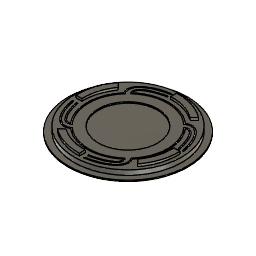
button (Autodesk Fusion 360 design; units mm, degrees)
Autodesk Fusion 360 part; units mm, degrees
note: some values were not read from the file. Set by a fixed rule: which sketch regions a step uses.
sketch "Sketch8" plane through (0, 0, 0) normal (0, 0, 1) x (1, 0, 0)
  circle A0 centre (0, 0) radius 40
  circle A1 centre (-48, 0) radius 2
  circle A2 centre (-48, 0) radius 4
  circle A3 centre (0, 0) radius 48 construction
  line L0 (-39.5395, 39.5395) -> (0, 0) construction
  line L1 (0, 0) -> (-68, 0) construction
  line L2 (-49.7486, 0.9707) -> (-47.9713, 22.4598) construction
  line L3 (-47.9713, 22.4598) -> (-35.9328, 37.1294) construction
  line L4 (-35.9328, 37.1294) -> (-26.8347, 29.6631) construction
  spline S0 degree 3 poles (-49.7486, 0.9707) (-47.9713, 22.4598) (-35.9328, 37.1294) (-26.8347, 29.6631) knots 0 0 0 0 1 1 1 1
  line L5 (-47.2849, 1.8678) -> (-43.4766, 23.129) construction
  line L6 (-43.4766, 23.129) -> (-35.7051, 32.0803) construction
  line L7 (-35.7051, 32.0803) -> (-29.6631, 26.8347) construction
  spline S1 degree 3 poles (-47.2849, 1.8678) (-43.4766, 23.129) (-35.7051, 32.0803) (-29.6631, 26.8347) knots 0 0 0 0 1 1 1 1
  dimension "d92" = 80
  dimension "d93" = 4
  dimension "d94" = 2
  dimension "d95" = 8
  dimension "d96" = 68
  dimension "d97" = 45
  dimension "d100" = 4
  dimension "d101" = 90
  dimension "d102" = 90
  dimension "d103" = 5.0542
  dimension "d104" = 2
  constraint coincident A0.centre A3.centre
  constraint horizontal A0.centre A1.centre
  constraint coincident A1.centre A3
  constraint horizontal L1
  constraint coincident A0 L7.end
  constraint coincident A0 L4.end
  constraint coincident A1 L2.start
  constraint coincident A1 L5.start
  constraint coincident A3 L6.end
  measures "d92" diameter of A0
  measures "d93" diameter of A1
  measures "d94" distance of A1
  measures "d96" distance of A0.centre L1.end
  measures "d97" angle of L0 L1
  measures "d100" distance of L4.end L7.end
  measures "d101" angle of L3 L4
  measures "d102" angle of L6 L7
  measures "d103" distance of L3.end L6.end
  measures "d104" distance of L0 L7.end
extrude "Extrude11" add sketch "Sketch8" along normal blind 6 contours A0 makes body 1
extrude "Extrude16" add sketch "Sketch8" along normal blind 6 separate body contours A0 A2 S0 S1 makes body 2
extrude "Extrude18" add sketch "Sketch8" along normal blind 6 contours A1 A2 S0 S1 | A1 A2 S0 S1 | A1 bodies 2
pattern_circular "C-Pattern2" count 4 over 360 about axis through (0, 0, 1.75) along (0, 0, 1) of "Extrude16", "Extrude18" makes body 3 at (-6.6102, -49.0265, 2) makes body 4 at (49.0265, -6.6102, 2) makes body 5 at (9.3884, 48.4723, 4)
sketch "Sketch11" plane through (0, 0, 6) normal (0, 0, 1) x (-1, 0, 0)
  circle A0 centre (0, 0) radius 40
  circle A1 centre (0, 0) radius 38
  dimension "d126" = 76
  constraint concentric A0 A1
  measures "d126" diameter of A1
sketch "Sketch15" plane through (0, 0, 0) normal (0, 0, -1) x (1, 0, 0)
  circle A0 centre (0, 0) radius 40
  circle A1 centre (0, 0) radius 54.5
  circle A2 centre (0, 0) radius 41.2
  spline S0 degree 3 poles (3.7237, -49.461) (23.6891, -46.9339) (36.806, -35.5387) (29.6631, -26.8347) knots 0.043317 0.043317 0.043317 0.043317 1 1 1 1
  spline S1 degree 3 poles (3.8491, -46.9116) (23.6813, -42.9865) (31.9143, -35.5139) (26.8347, -29.6631) knots 0.031644 0.031644 0.031644 0.031644 1 1 1 1
  spline S2 degree 3 poles (46.9116, 3.8491) (42.9865, 23.6813) (35.5139, 31.9143) (29.6631, 26.8347) knots 0.031644 0.031644 0.031644 0.031644 1 1 1 1
  spline S3 degree 3 poles (49.461, 3.7237) (46.9339, 23.6891) (35.5387, 36.806) (26.8347, 29.6631) knots 0.043317 0.043317 0.043317 0.043317 1 1 1 1
  arc A3 (46.9116, 3.8491) -> (49.461, 3.7237) centre (48, 0) ccw
  spline S4 degree 3 poles (3.8491, -46.9116) (23.6813, -42.9865) (31.9143, -35.5139) (26.8347, -29.6631) knots 0.031644 0.031644 0.031644 0.031644 1 1 1 1
  arc A4 (3.8491, -46.9116) -> (3.7237, -49.461) centre (0, -48) ccw
  spline S5 degree 3 poles (3.7237, -49.461) (23.6891, -46.9339) (36.806, -35.5387) (29.6631, -26.8347) knots 0.043317 0.043317 0.043317 0.043317 1 1 1 1
  arc A5 (26.8347, -29.6631) -> (29.6631, -26.8347) centre (0, 0) ccw
  arc A6 (-46.9116, -3.8491) -> (-49.461, -3.7237) centre (-48, 0) ccw
  spline S6 degree 3 poles (-46.9116, -3.8491) (-42.9865, -23.6813) (-35.5139, -31.9143) (-29.6631, -26.8347) knots 0.031644 0.031644 0.031644 0.031644 1 1 1 1
  spline S7 degree 3 poles (-49.461, -3.7237) (-46.9339, -23.6891) (-35.5387, -36.806) (-26.8347, -29.6631) knots 0.043317 0.043317 0.043317 0.043317 1 1 1 1
  spline S8 degree 3 poles (-3.7237, 49.461) (-23.6891, 46.9339) (-36.806, 35.5387) (-29.6631, 26.8347) knots 0.043317 0.043317 0.043317 0.043317 1 1 1 1
  spline S9 degree 3 poles (-3.8491, 46.9116) (-23.6813, 42.9865) (-31.9143, 35.5139) (-26.8347, 29.6631) knots 0.031644 0.031644 0.031644 0.031644 1 1 1 1
  arc A7 (-3.8491, 46.9116) -> (-3.7237, 49.461) centre (0, 48) ccw
  arc A8 (-2.6359, 43.5347) -> (-3.3902, 43.6926) centre (-3.2459, 42.5013) ccw
  arc A9 (-5.0161, 50.5234) -> (-4.2204, 51.0125) centre (-5.1971, 51.7097) ccw
  arc A10 (44.9096, 4.1704) -> (45.3659, 5.3977) centre (44.1951, 5.1345) ccw
  arc A11 (50.4825, 5.0583) -> (50.9808, 4.2495) centre (51.6699, 5.2319) ccw
  arc A12 (5.0569, -50.486) -> (4.2495, -50.9837) centre (5.2316, -51.6732) ccw
  arc A13 (4.1719, -44.9087) -> (5.3984, -45.3653) centre (5.1361, -44.1943) ccw
  spline S10 degree 3 poles (-50.566, -4.5228) (-49.2121, -14.4065) (-45.7541, -22.6133) (-41.369, -27.6472) (-39.0131, -30.3518) (-36.3616, -32.1693) (-33.542, -32.6861) (-31.191, -33.1171) (-28.7542, -32.5715) (-26.5965, -30.9961) (-26.4205, -30.8676) (-26.2461, -30.7325) (-26.0734, -30.5907) knots 0.053517 0.053517 0.053517 0.053517 0.521659 0.521659 0.521659 0.77317 0.77317 0.77317 0.982893 0.982893 0.982893 1 1 1 1
  arc A14 (-45.5388, -4.5807) -> (-50.566, -4.5228) centre (-48, 0) ccw
  spline S11 degree 3 poles (-45.5388, -4.5807) (-43.7792, -13.0486) (-41.3441, -19.2391) (-38.8101, -22.9312) (-37.3314, -25.0858) (-35.8297, -26.3571) (-34.5346, -26.8443) (-33.5151, -27.2279) (-32.632, -27.1972) (-31.6708, -26.744) (-31.2743, -26.557) (-30.8658, -26.2897) (-30.4498, -25.9285) knots 0.04768 0.04768 0.04768 0.04768 0.474261 0.474261 0.474261 0.723202 0.723202 0.723202 0.919177 0.919177 0.919177 1 1 1 1
  spline S12 degree 3 poles (-4.5807, 45.5388) (-13.0486, 43.7792) (-19.2391, 41.3441) (-22.9312, 38.8101) (-25.0858, 37.3314) (-26.3571, 35.8297) (-26.8443, 34.5346) (-27.2279, 33.5151) (-27.1972, 32.632) (-26.744, 31.6708) (-26.557, 31.2743) (-26.2897, 30.8658) (-25.9285, 30.4498) knots 0.04768 0.04768 0.04768 0.04768 0.474261 0.474261 0.474261 0.723202 0.723202 0.723202 0.919177 0.919177 0.919177 1 1 1 1
  arc A15 (-4.5807, 45.5388) -> (-4.5228, 50.566) centre (0, 48) ccw
  spline S13 degree 3 poles (-4.5228, 50.566) (-14.4065, 49.2121) (-22.6133, 45.7541) (-27.6472, 41.369) (-30.3518, 39.0131) (-32.1693, 36.3616) (-32.6861, 33.542) (-33.1171, 31.191) (-32.5715, 28.7542) (-30.9961, 26.5965) (-30.8676, 26.4205) (-30.7325, 26.2461) (-30.5907, 26.0734) knots 0.053517 0.053517 0.053517 0.053517 0.521659 0.521659 0.521659 0.77317 0.77317 0.77317 0.982893 0.982893 0.982893 1 1 1 1
  spline S14 degree 3 poles (45.5388, 4.5807) (43.7792, 13.0486) (41.3441, 19.2391) (38.8101, 22.9312) (37.3314, 25.0858) (35.8297, 26.3571) (34.5346, 26.8443) (33.5151, 27.2279) (32.632, 27.1972) (31.6708, 26.744) (31.2743, 26.557) (30.8658, 26.2897) (30.4498, 25.9285) knots 0.04768 0.04768 0.04768 0.04768 0.474261 0.474261 0.474261 0.723202 0.723202 0.723202 0.919177 0.919177 0.919177 1 1 1 1
  arc A16 (45.5388, 4.5807) -> (50.566, 4.5228) centre (48, 0) ccw
  spline S15 degree 3 poles (50.566, 4.5228) (49.2121, 14.4065) (45.7541, 22.6133) (41.369, 27.6472) (39.0131, 30.3518) (36.3616, 32.1693) (33.542, 32.6861) (31.191, 33.1171) (28.7542, 32.5715) (26.5965, 30.9961) (26.4205, 30.8676) (26.2461, 30.7325) (26.0734, 30.5907) knots 0.053517 0.053517 0.053517 0.053517 0.521659 0.521659 0.521659 0.77317 0.77317 0.77317 0.982893 0.982893 0.982893 1 1 1 1
  spline S16 degree 3 poles (4.5228, -50.566) (14.4065, -49.2121) (22.6133, -45.7541) (27.6472, -41.369) (30.3518, -39.0131) (32.1693, -36.3616) (32.6861, -33.542) (33.1171, -31.191) (32.5715, -28.7542) (30.9961, -26.5965) (30.8676, -26.4205) (30.7325, -26.2461) (30.5907, -26.0734) knots 0.053517 0.053517 0.053517 0.053517 0.521659 0.521659 0.521659 0.77317 0.77317 0.77317 0.982893 0.982893 0.982893 1 1 1 1
  arc A17 (4.5807, -45.5388) -> (4.5228, -50.566) centre (0, -48) ccw
  spline S17 degree 3 poles (4.5807, -45.5388) (13.0486, -43.7792) (19.2391, -41.3441) (22.9312, -38.8101) (25.0858, -37.3314) (26.3571, -35.8297) (26.8443, -34.5346) (27.2279, -33.5151) (27.1972, -32.632) (26.744, -31.6708) (26.557, -31.2743) (26.2897, -30.8658) (25.9285, -30.4498) knots 0.04768 0.04768 0.04768 0.04768 0.474261 0.474261 0.474261 0.723202 0.723202 0.723202 0.919177 0.919177 0.919177 1 1 1 1
  dimension "d155" = 109
  dimension "d156" = 82.4
  dimension "d167" = 1.2
  dimension "d168" = 1.2
  dimension "d169" = 1.2
  dimension "d170" = 1.2
  dimension "d171" = 1.2
  dimension "d172" = 1.2
  dimension "d178" = 1.2
  dimension "d207" = 1.2
  dimension "d208" = 1.2
  constraint concentric A0 A1
  constraint concentric A0 A2
  measures "d155" diameter of A1
  measures "d156" diameter of A2
  measures "d167" radius of A8
  measures "d168" radius of A9
  measures "d169" radius of A10
  measures "d170" radius of A11
  measures "d171" radius of A12
  measures "d172" radius of A13
extrude "Extrude23" add sketch "Sketch15" against normal blind 6 separate body makes body 6
combine "Combine4" operation add target body 1 tool bodies 3 4 5 2 6 makes body 7 at (46.2947, 10.9613, 0)
sketch "Sketch18" plane through (0, 0, 6) normal (0, 0, 1) x (-1, 0, 0)
  spline S0 degree 3 poles (50.566, -4.5228) (49.2121, -14.4065) (45.7541, -22.6133) (41.369, -27.6472) (39.0131, -30.3518) (36.3616, -32.1693) (33.542, -32.6861) (31.2997, -33.0972) (28.9795, -32.6199) (26.8976, -31.2084) knots 0.053517 0.053517 0.053517 0.053517 0.521659 0.521659 0.521659 0.77317 0.77317 0.77317 0.97319 0.97319 0.97319 0.97319
  arc A0 (-31.4398, 26.6266) -> (-31.2084, -26.8976) centre (0, 0) ccw
  spline S1 degree 3 poles (31.4398, -26.6266) (31.5172, -26.6688) (31.5942, -26.7079) (31.6708, -26.744) (32.632, -27.1972) (33.5151, -27.2279) (34.5346, -26.8443) (35.8297, -26.3571) (37.3314, -25.0858) (38.8101, -22.9312) (41.3441, -19.2391) (43.7792, -13.0486) (45.5388, -4.5807) knots -0.934786 -0.934786 -0.934786 -0.934786 -0.919177 -0.919177 -0.919177 -0.723202 -0.723202 -0.723202 -0.474261 -0.474261 -0.474261 -0.04768 -0.04768 -0.04768 -0.04768
  arc A1 (50.566, -4.5228) -> (45.5388, -4.5807) centre (48, 0) ccw
  circle A2 centre (48, 0) radius 6
  circle A3 centre (0, 0) radius 54.5
  arc A4 (4.5228, 50.566) -> (4.5807, 45.5388) centre (0, 48) ccw
  spline S2 degree 3 poles (4.5228, 50.566) (14.4065, 49.2121) (22.6133, 45.7541) (27.6472, 41.369) (30.3518, 39.0131) (32.1693, 36.3616) (32.6861, 33.542) (33.0972, 31.2997) (32.6199, 28.9795) (31.2084, 26.8976) knots 0.053517 0.053517 0.053517 0.053517 0.521659 0.521659 0.521659 0.77317 0.77317 0.77317 0.97319 0.97319 0.97319 0.97319
  spline S3 degree 3 poles (26.6266, 31.4398) (26.6688, 31.5172) (26.7079, 31.5942) (26.744, 31.6708) (27.1972, 32.632) (27.2279, 33.5151) (26.8443, 34.5346) (26.3571, 35.8297) (25.0858, 37.3314) (22.9312, 38.8101) (19.2391, 41.3441) (13.0486, 43.7792) (4.5807, 45.5388) knots -0.934786 -0.934786 -0.934786 -0.934786 -0.919177 -0.919177 -0.919177 -0.723202 -0.723202 -0.723202 -0.474261 -0.474261 -0.474261 -0.04768 -0.04768 -0.04768 -0.04768
  spline S4 degree 3 poles (-4.9578, -50.5049) (-14.6472, -49.1102) (-22.6873, -45.6896) (-27.6472, -41.369) (-30.3518, -39.0131) (-32.1693, -36.3616) (-32.6861, -33.542) (-33.0972, -31.2997) (-32.6199, -28.9795) (-31.2084, -26.8976) knots 0.060402 0.060402 0.060402 0.060402 0.521659 0.521659 0.521659 0.77317 0.77317 0.77317 0.97319 0.97319 0.97319 0.97319
  spline S5 degree 3 poles (-31.4398, 26.6266) (-31.5172, 26.6688) (-31.5942, 26.7079) (-31.6708, 26.744) (-32.632, 27.1972) (-33.5151, 27.2279) (-34.5346, 26.8443) (-35.8297, 26.3571) (-37.3314, 25.0858) (-38.8101, 22.9312) (-41.2659, 19.3529) (-43.6289, 13.428) (-45.3742, 5.3575) knots -0.934786 -0.934786 -0.934786 -0.934786 -0.919177 -0.919177 -0.919177 -0.723202 -0.723202 -0.723202 -0.474261 -0.474261 -0.474261 -0.060835 -0.060835 -0.060835 -0.060835
  arc A5 (-45.3742, 5.3575) -> (-45.0133, 4.2567) centre (-44.1951, 5.1345) ccw
  arc A6 (-50.8748, 4.3331) -> (-45.0133, 4.2567) centre (-48, 0) ccw
  arc A7 (-50.8748, 4.3331) -> (-50.5094, 4.9263) centre (-51.6699, 5.2319) ccw
  spline S6 degree 3 poles (-50.5094, 4.9263) (-49.1175, 14.6298) (-45.6942, 22.6819) (-41.369, 27.6472) (-39.0131, 30.3518) (-36.3616, 32.1693) (-33.542, 32.6861) (-31.2997, 33.0972) (-28.9795, 32.6199) (-26.8976, 31.2084) knots 0.059903 0.059903 0.059903 0.059903 0.521659 0.521659 0.521659 0.77317 0.77317 0.77317 0.97319 0.97319 0.97319 0.97319
  arc A8 (26.6266, 31.4398) -> (-26.8976, 31.2084) centre (0, 0) ccw
  arc A9 (31.4398, -26.6266) -> (31.2084, 26.8976) centre (0, 0) ccw
  arc A10 (-26.6266, -31.4398) -> (26.8976, -31.2084) centre (0, 0) ccw
  spline S7 degree 3 poles (-26.6266, -31.4398) (-26.6688, -31.5172) (-26.7079, -31.5942) (-26.744, -31.6708) (-27.1972, -32.632) (-27.2279, -33.5151) (-26.8443, -34.5346) (-26.3571, -35.8297) (-25.0858, -37.3314) (-22.9312, -38.8101) (-19.2391, -41.3441) (-13.0486, -43.7792) (-4.5807, -45.5388) knots -0.934786 -0.934786 -0.934786 -0.934786 -0.919177 -0.919177 -0.919177 -0.723202 -0.723202 -0.723202 -0.474261 -0.474261 -0.474261 -0.04768 -0.04768 -0.04768 -0.04768
  arc A11 (-4.3245, -50.8876) -> (-4.5807, -45.5388) centre (0, -48) ccw
  arc A12 (-4.3245, -50.8876) -> (-4.9578, -50.5049) centre (-5.2316, -51.6732) ccw
  dimension "d185" = 12
  constraint concentric A1 A2
  measures "d185" diameter of A2
extrude "Extrude26" add sketch "Sketch18" against normal blind 6 contours S0 S1 A1 A2 | S0 S1 A1 A2 bodies 1 7
pattern_circular "C-Pattern5" count 4 over 360 about axis through (0, 0, 1.75) along (0, 0, 1) of "Extrude26"
sketch "Sketch19" plane through (0, 0, 6) normal (0, 0, 1) x (-1, 0, 0)
  spline S0 degree 3 poles (-46.5038, 5.8105) (-42.4857, 24.22) (-35.3171, 31.7435) (-29.6631, 26.8347) knots 0.064208 0.064208 0.064208 0.064208 1 1 1 1
  arc A0 (-29.6631, 26.8347) -> (-29.6631, -26.8347) centre (0, 0) ccw
  spline S1 degree 3 poles (-29.6631, -26.8347) (-36.5444, -35.2199) (-24.6228, -46.1028) (-5.8891, -49.1482) knots -1 -1 -1 -1 -0.078355 -0.078355 -0.078355 -0.078355
  spline S2 degree 3 poles (-5.8105, -46.5038) (-24.22, -42.4857) (-31.7435, -35.3171) (-26.8347, -29.6631) knots 0.064208 0.064208 0.064208 0.064208 1 1 1 1
  arc A1 (-26.8347, -29.6631) -> (26.8347, -29.6631) centre (0, 0) ccw
  spline S3 degree 3 poles (26.8347, -29.6631) (35.2199, -36.5444) (46.1028, -24.6228) (49.1482, -5.8891) knots -1 -1 -1 -1 -0.078355 -0.078355 -0.078355 -0.078355
  arc A2 (49.1482, -5.8891) -> (50.4263, -5.4875) centre (48, 0) ccw
  spline S4 degree 3 poles (50.4263, -5.4875) (48.9827, -14.9399) (45.6106, -22.778) (41.369, -27.6472) (39.0131, -30.3518) (36.3616, -32.1693) (33.542, -32.6861) (31.2997, -33.0972) (28.9795, -32.6199) (26.8976, -31.2084) knots 0.068835 0.068835 0.068835 0.068835 0.521659 0.521659 0.521659 0.77317 0.77317 0.77317 0.97319 0.97319 0.97319 0.97319
  circle A3 centre (0, 0) radius 54.5
  spline S5 degree 3 poles (31.4398, -26.6266) (31.5172, -26.6688) (31.5942, -26.7079) (31.6708, -26.744) (32.632, -27.1972) (33.5151, -27.2279) (34.5346, -26.8443) (35.8297, -26.3571) (37.3314, -25.0858) (38.8101, -22.9312) (41.2625, -19.3579) (43.6223, -13.4446) (45.3669, -5.3913) knots -0.934786 -0.934786 -0.934786 -0.934786 -0.919177 -0.919177 -0.919177 -0.723202 -0.723202 -0.723202 -0.474261 -0.474261 -0.474261 -0.061414 -0.061414 -0.061414 -0.061414
  arc A4 (45.3669, -5.3913) -> (46.5038, -5.8105) centre (48, 0) ccw
  spline S6 degree 3 poles (46.5038, -5.8105) (42.4857, -24.22) (35.3171, -31.7435) (29.6631, -26.8347) knots 0.064208 0.064208 0.064208 0.064208 1 1 1 1
  arc A5 (29.6631, -26.8347) -> (29.6631, 26.8347) centre (0, 0) ccw
  spline S7 degree 3 poles (29.6631, 26.8347) (36.5444, 35.2199) (24.6228, 46.1028) (5.8891, 49.1482) knots -1 -1 -1 -1 -0.078355 -0.078355 -0.078355 -0.078355
  arc A6 (5.3913, 45.3669) -> (5.8105, 46.5038) centre (0, 48) ccw
  arc A7 (-31.4398, 26.6266) -> (-31.2084, -26.8976) centre (0, 0) ccw
  spline S8 degree 3 poles (5.8105, 46.5038) (24.22, 42.4857) (31.7435, 35.3171) (26.8347, 29.6631) knots 0.064208 0.064208 0.064208 0.064208 1 1 1 1
  arc A8 (26.8347, 29.6631) -> (-26.8347, 29.6631) centre (0, 0) ccw
  spline S9 degree 3 poles (-26.8347, 29.6631) (-35.2199, 36.5444) (-46.1028, 24.6228) (-49.1482, 5.8891) knots -1 -1 -1 -1 -0.078355 -0.078355 -0.078355 -0.078355
  circle A9 centre (0, 0) radius 54.5
  circle A10 centre (0, 0) radius 60.5
  spline S10 degree 3 poles (26.6266, 31.4398) (26.6688, 31.5172) (26.7079, 31.5942) (26.744, 31.6708) (27.1972, 32.632) (27.2279, 33.5151) (26.8443, 34.5346) (26.3571, 35.8297) (25.0858, 37.3314) (22.9312, 38.8101) (19.3579, 41.2625) (13.4446, 43.6223) (5.3913, 45.3669) knots -0.934786 -0.934786 -0.934786 -0.934786 -0.919177 -0.919177 -0.919177 -0.723202 -0.723202 -0.723202 -0.474261 -0.474261 -0.474261 -0.061414 -0.061414 -0.061414 -0.061414
  spline S11 degree 3 poles (5.4875, 50.4263) (14.9399, 48.9827) (22.778, 45.6106) (27.6472, 41.369) (30.3518, 39.0131) (32.1693, 36.3616) (32.6861, 33.542) (33.0972, 31.2997) (32.6199, 28.9795) (31.2084, 26.8976) knots 0.068835 0.068835 0.068835 0.068835 0.521659 0.521659 0.521659 0.77317 0.77317 0.77317 0.97319 0.97319 0.97319 0.97319
  arc A11 (31.4398, -26.6266) -> (31.2084, 26.8976) centre (0, 0) ccw
  arc A12 (5.8891, 49.1482) -> (5.4875, 50.4263) centre (0, 48) ccw
  arc A13 (-26.6266, -31.4398) -> (26.8976, -31.2084) centre (0, 0) ccw
  spline S12 degree 3 poles (-5.4875, -50.4263) (-14.9399, -48.9827) (-22.778, -45.6106) (-27.6472, -41.369) (-30.3518, -39.0131) (-32.1693, -36.3616) (-32.6861, -33.542) (-33.0972, -31.2997) (-32.6199, -28.9795) (-31.2084, -26.8976) knots 0.068835 0.068835 0.068835 0.068835 0.521659 0.521659 0.521659 0.77317 0.77317 0.77317 0.97319 0.97319 0.97319 0.97319
  spline S13 degree 3 poles (-31.4398, 26.6266) (-31.5172, 26.6688) (-31.5942, 26.7079) (-31.6708, 26.744) (-32.632, 27.1972) (-33.5151, 27.2279) (-34.5346, 26.8443) (-35.8297, 26.3571) (-37.3314, 25.0858) (-38.8101, 22.9312) (-41.2625, 19.3579) (-43.6223, 13.4446) (-45.3669, 5.3913) knots -0.934786 -0.934786 -0.934786 -0.934786 -0.919177 -0.919177 -0.919177 -0.723202 -0.723202 -0.723202 -0.474261 -0.474261 -0.474261 -0.061414 -0.061414 -0.061414 -0.061414
  arc A14 (-45.3669, 5.3913) -> (-46.5038, 5.8105) centre (-48, 0) ccw
  arc A15 (-5.8891, -49.1482) -> (-5.4875, -50.4263) centre (0, -48) ccw
  arc A16 (-5.3913, -45.3669) -> (-5.8105, -46.5038) centre (0, -48) ccw
  spline S14 degree 3 poles (-26.6266, -31.4398) (-26.6688, -31.5172) (-26.7079, -31.5942) (-26.744, -31.6708) (-27.1972, -32.632) (-27.2279, -33.5151) (-26.8443, -34.5346) (-26.3571, -35.8297) (-25.0858, -37.3314) (-22.9312, -38.8101) (-19.3579, -41.2625) (-13.4446, -43.6223) (-5.3913, -45.3669) knots -0.934786 -0.934786 -0.934786 -0.934786 -0.919177 -0.919177 -0.919177 -0.723202 -0.723202 -0.723202 -0.474261 -0.474261 -0.474261 -0.061414 -0.061414 -0.061414 -0.061414
  spline S15 degree 3 poles (-50.4263, 5.4875) (-48.9827, 14.9399) (-45.6106, 22.778) (-41.369, 27.6472) (-39.0131, 30.3518) (-36.3616, 32.1693) (-33.542, 32.6861) (-31.2997, 33.0972) (-28.9795, 32.6199) (-26.8976, 31.2084) knots 0.068835 0.068835 0.068835 0.068835 0.521659 0.521659 0.521659 0.77317 0.77317 0.77317 0.97319 0.97319 0.97319 0.97319
  arc A17 (26.6266, 31.4398) -> (-26.8976, 31.2084) centre (0, 0) ccw
  arc A18 (-49.1482, 5.8891) -> (-50.4263, 5.4875) centre (-48, 0) ccw
  dimension "d190" = 6
extrude "Extrude27" add sketch "Sketch19" against normal blind 1.2 contours A10 bodies 1
sketch "Sketch20" plane through (0, 0, 0) normal (0, 0, -1) x (1, 0, 0)
  spline S0 degree 3 poles (-26.8976, -31.2084) (-28.9795, -32.6199) (-31.2997, -33.0972) (-33.542, -32.6861) (-36.3616, -32.1693) (-39.0131, -30.3518) (-41.369, -27.6472) (-45.6106, -22.778) (-48.9827, -14.9399) (-50.4263, -5.4875) knots -0.97319 -0.97319 -0.97319 -0.97319 -0.77317 -0.77317 -0.77317 -0.521659 -0.521659 -0.521659 -0.068835 -0.068835 -0.068835 -0.068835
  arc A0 (-50.4263, -5.4875) -> (-49.1482, -5.8891) centre (-48, 0) ccw
  spline S1 degree 3 poles (-49.1482, -5.8891) (-46.1028, -24.6228) (-35.2199, -36.5444) (-26.8347, -29.6631) knots 0.078355 0.078355 0.078355 0.078355 1 1 1 1
  arc A1 (-26.8347, -29.6631) -> (26.8347, -29.6631) centre (0, 0) ccw
  spline S2 degree 3 poles (5.8105, -46.5038) (24.22, -42.4857) (31.7435, -35.3171) (26.8347, -29.6631) knots 0.064208 0.064208 0.064208 0.064208 1 1 1 1
  spline S3 degree 3 poles (5.8891, -49.1482) (24.6228, -46.1028) (36.5444, -35.2199) (29.6631, -26.8347) knots 0.078355 0.078355 0.078355 0.078355 1 1 1 1
  arc A2 (29.6631, -26.8347) -> (29.6631, 26.8347) centre (0, 0) ccw
  spline S4 degree 3 poles (46.5038, 5.8105) (42.4857, 24.22) (35.3171, 31.7435) (29.6631, 26.8347) knots 0.064208 0.064208 0.064208 0.064208 1 1 1 1
  circle A3 centre (0, 0) radius 54.5
  arc A4 (-5.4875, 50.4263) -> (-5.8891, 49.1482) centre (0, 48) ccw
  spline S5 degree 3 poles (-5.8891, 49.1482) (-24.6228, 46.1028) (-36.5444, 35.2199) (-29.6631, 26.8347) knots 0.078355 0.078355 0.078355 0.078355 1 1 1 1
  arc A5 (-29.6631, 26.8347) -> (-29.6631, -26.8347) centre (0, 0) ccw
  spline S6 degree 3 poles (-46.5038, -5.8105) (-42.4857, -24.22) (-35.3171, -31.7435) (-29.6631, -26.8347) knots 0.064208 0.064208 0.064208 0.064208 1 1 1 1
  arc A6 (-46.5038, -5.8105) -> (-45.3669, -5.3913) centre (-48, 0) ccw
  spline S7 degree 3 poles (-45.3669, -5.3913) (-43.6223, -13.4446) (-41.2625, -19.3579) (-38.8101, -22.9312) (-37.3314, -25.0858) (-35.8297, -26.3571) (-34.5346, -26.8443) (-33.5151, -27.2279) (-32.632, -27.1972) (-31.6708, -26.744) (-31.5942, -26.7079) (-31.5172, -26.6688) (-31.4398, -26.6266) knots 0.061414 0.061414 0.061414 0.061414 0.474261 0.474261 0.474261 0.723202 0.723202 0.723202 0.919177 0.919177 0.919177 0.934786 0.934786 0.934786 0.934786
  spline S8 degree 3 poles (49.1482, 5.8891) (46.1028, 24.6228) (35.2199, 36.5444) (26.8347, 29.6631) knots 0.078355 0.078355 0.078355 0.078355 1 1 1 1
  arc A7 (26.8347, 29.6631) -> (-26.8347, 29.6631) centre (0, 0) ccw
  spline S9 degree 3 poles (-5.8105, 46.5038) (-24.22, 42.4857) (-31.7435, 35.3171) (-26.8347, 29.6631) knots 0.064208 0.064208 0.064208 0.064208 1 1 1 1
  arc A8 (-5.8105, 46.5038) -> (-5.3913, 45.3669) centre (0, 48) ccw
  arc A9 (-26.8976, -31.2084) -> (26.6266, -31.4398) centre (0, 0) ccw
  circle A10 centre (0, 0) radius 48 construction
  circle A11 centre (0, 0) radius 51
  circle A12 centre (0, 0) radius 45
  line L0 (26.4027, 36.4403) -> (30.8631, 40.6014)
  line L1 (-1.7183, 44.9672) -> (-1.7183, 50.971)
  spline S10 degree 3 poles (-5.3913, 45.3669) (-13.4446, 43.6223) (-19.3579, 41.2625) (-22.9312, 38.8101) (-25.0858, 37.3314) (-26.3571, 35.8297) (-26.8443, 34.5346) (-27.2279, 33.5151) (-27.1972, 32.632) (-26.744, 31.6708) (-26.7079, 31.5942) (-26.6688, 31.5172) (-26.6266, 31.4398) knots 0.061414 0.061414 0.061414 0.061414 0.474261 0.474261 0.474261 0.723202 0.723202 0.723202 0.919177 0.919177 0.919177 0.934786 0.934786 0.934786 0.934786
  arc A13 (-31.2084, 26.8976) -> (-31.4398, -26.6266) centre (0, 0) ccw
  spline S11 degree 3 poles (-31.2084, 26.8976) (-32.6199, 28.9795) (-33.0972, 31.2997) (-32.6861, 33.542) (-32.1693, 36.3616) (-30.3518, 39.0131) (-27.6472, 41.369) (-22.778, 45.6106) (-14.9399, 48.9827) (-5.4875, 50.4263) knots -0.97319 -0.97319 -0.97319 -0.97319 -0.77317 -0.77317 -0.77317 -0.521659 -0.521659 -0.521659 -0.068835 -0.068835 -0.068835 -0.068835
  spline S12 degree 3 poles (5.3913, -45.3669) (13.4446, -43.6223) (19.3579, -41.2625) (22.9312, -38.8101) (25.0858, -37.3314) (26.3571, -35.8297) (26.8443, -34.5346) (27.2279, -33.5151) (27.1972, -32.632) (26.744, -31.6708) (26.7079, -31.5942) (26.6688, -31.5172) (26.6266, -31.4398) knots 0.061414 0.061414 0.061414 0.061414 0.474261 0.474261 0.474261 0.723202 0.723202 0.723202 0.919177 0.919177 0.919177 0.934786 0.934786 0.934786 0.934786
  arc A14 (5.8105, -46.5038) -> (5.3913, -45.3669) centre (0, -48) ccw
  arc A15 (5.4875, -50.4263) -> (5.8891, -49.1482) centre (0, -48) ccw
  arc A16 (46.5038, 5.8105) -> (45.3669, 5.3913) centre (48, 0) ccw
  spline S13 degree 3 poles (45.3669, 5.3913) (43.6223, 13.4446) (41.2625, 19.3579) (38.8101, 22.9312) (37.3314, 25.0858) (35.8297, 26.3571) (34.5346, 26.8443) (33.5151, 27.2279) (32.632, 27.1972) (31.6708, 26.744) (31.5942, 26.7079) (31.5172, 26.6688) (31.4398, 26.6266) knots 0.061414 0.061414 0.061414 0.061414 0.474261 0.474261 0.474261 0.723202 0.723202 0.723202 0.919177 0.919177 0.919177 0.934786 0.934786 0.934786 0.934786
  arc A17 (31.2084, -26.8976) -> (31.4398, 26.6266) centre (0, 0) ccw
  spline S14 degree 3 poles (31.2084, -26.8976) (32.6199, -28.9795) (33.0972, -31.2997) (32.6861, -33.542) (32.1693, -36.3616) (30.3518, -39.0131) (27.6472, -41.369) (22.778, -45.6106) (14.9399, -48.9827) (5.4875, -50.4263) knots -0.97319 -0.97319 -0.97319 -0.97319 -0.77317 -0.77317 -0.77317 -0.521659 -0.521659 -0.521659 -0.068835 -0.068835 -0.068835 -0.068835
  arc A18 (50.4263, 5.4875) -> (49.1482, 5.8891) centre (48, 0) ccw
  arc A19 (26.8976, 31.2084) -> (-26.6266, 31.4398) centre (0, 0) ccw
  spline S15 degree 3 poles (26.8976, 31.2084) (28.9795, 32.6199) (31.2997, 33.0972) (33.542, 32.6861) (36.3616, 32.1693) (39.0131, 30.3518) (41.369, 27.6472) (45.6106, 22.778) (48.9827, 14.9399) (50.4263, 5.4875) knots -0.97319 -0.97319 -0.97319 -0.97319 -0.77317 -0.77317 -0.77317 -0.521659 -0.521659 -0.521659 -0.068835 -0.068835 -0.068835 -0.068835
  dimension "d194" = 96
  dimension "d204" = 3
  dimension "d205" = -3
  constraint coincident A1.centre A2.centre
  constraint coincident A12 L0.start
  constraint coincident A11 L0.end
  constraint coincident A12 L1.start
  constraint coincident A11 L1.end
  constraint vertical L1
  measures "d194" diameter of A10
extrude "Extrude28" add sketch "Sketch20" along normal blind 2.4 contours A11 A12 L0 L1 bodies 1
pattern_circular "C-Pattern6" count 4 over 360 about axis through (0, 0, 1.75) along (0, 0, 1) of "Extrude28"
sketch "Sketch21" plane through (0, 0, 0) normal (0, 0, -1) x (1, 0, 0)
  spline S0 degree 3 poles (-26.8976, -31.2084) (-28.9795, -32.6199) (-31.2997, -33.0972) (-33.542, -32.6861) (-36.3616, -32.1693) (-39.0131, -30.3518) (-41.369, -27.6472) (-45.6106, -22.778) (-48.9827, -14.9399) (-50.4263, -5.4875) knots -0.97319 -0.97319 -0.97319 -0.97319 -0.77317 -0.77317 -0.77317 -0.521659 -0.521659 -0.521659 -0.068835 -0.068835 -0.068835 -0.068835
  arc A0 (-50.4263, -5.4875) -> (-49.1482, -5.8891) centre (-48, 0) ccw
  spline S1 degree 3 poles (-49.1482, -5.8891) (-46.1028, -24.6228) (-35.2199, -36.5444) (-26.8347, -29.6631) knots 0.078355 0.078355 0.078355 0.078355 1 1 1 1
  arc A1 (-26.8347, -29.6631) -> (26.8347, -29.6631) centre (0, 0) ccw
  spline S2 degree 3 poles (5.8105, -46.5038) (24.22, -42.4857) (31.7435, -35.3171) (26.8347, -29.6631) knots 0.064208 0.064208 0.064208 0.064208 1 1 1 1
  spline S3 degree 3 poles (5.8891, -49.1482) (24.6228, -46.1028) (36.5444, -35.2199) (29.6631, -26.8347) knots 0.078355 0.078355 0.078355 0.078355 1 1 1 1
  arc A2 (29.6631, -26.8347) -> (29.6631, 26.8347) centre (0, 0) ccw
  spline S4 degree 3 poles (46.5038, 5.8105) (42.4857, 24.22) (35.3171, 31.7435) (29.6631, 26.8347) knots 0.064208 0.064208 0.064208 0.064208 1 1 1 1
  circle A3 centre (0, 0) radius 54.5
  arc A4 (-5.4875, 50.4263) -> (-5.8891, 49.1482) centre (0, 48) ccw
  spline S5 degree 3 poles (-5.8891, 49.1482) (-24.6228, 46.1028) (-36.5444, 35.2199) (-29.6631, 26.8347) knots 0.078355 0.078355 0.078355 0.078355 1 1 1 1
  arc A5 (-29.6631, 26.8347) -> (-29.6631, -26.8347) centre (0, 0) ccw
  spline S6 degree 3 poles (-46.5038, -5.8105) (-42.4857, -24.22) (-35.3171, -31.7435) (-29.6631, -26.8347) knots 0.064208 0.064208 0.064208 0.064208 1 1 1 1
  arc A6 (-46.5038, -5.8105) -> (-45.3669, -5.3913) centre (-48, 0) ccw
  spline S7 degree 3 poles (-45.3669, -5.3913) (-43.6223, -13.4446) (-41.2625, -19.3579) (-38.8101, -22.9312) (-37.3314, -25.0858) (-35.8297, -26.3571) (-34.5346, -26.8443) (-33.5151, -27.2279) (-32.632, -27.1972) (-31.6708, -26.744) (-31.5942, -26.7079) (-31.5172, -26.6688) (-31.4398, -26.6266) knots 0.061414 0.061414 0.061414 0.061414 0.474261 0.474261 0.474261 0.723202 0.723202 0.723202 0.919177 0.919177 0.919177 0.934786 0.934786 0.934786 0.934786
  spline S8 degree 3 poles (49.1482, 5.8891) (46.1028, 24.6228) (35.2199, 36.5444) (26.8347, 29.6631) knots 0.078355 0.078355 0.078355 0.078355 1 1 1 1
  arc A7 (26.8347, 29.6631) -> (-26.8347, 29.6631) centre (0, 0) ccw
  spline S9 degree 3 poles (-5.8105, 46.5038) (-24.22, 42.4857) (-31.7435, 35.3171) (-26.8347, 29.6631) knots 0.064208 0.064208 0.064208 0.064208 1 1 1 1
  arc A8 (-5.8105, 46.5038) -> (-5.3913, 45.3669) centre (0, 48) ccw
  arc A9 (-26.8976, -31.2084) -> (26.6266, -31.4398) centre (0, 0) ccw
  circle A10 centre (0, 0) radius 30
  arc A11 (26.4027, 36.4403) -> (-1.7183, 44.9672) centre (0, 0) ccw
  line L0 (-1.7183, 44.9672) -> (-1.7183, 50.971)
  arc A12 (30.8631, 40.6014) -> (-1.7183, 50.971) centre (0, 0) ccw
  line L1 (30.8631, 40.6014) -> (26.4027, 36.4403)
  arc A13 (-36.4403, 26.4027) -> (-44.9672, -1.7183) centre (0, 0) ccw
  line L2 (-44.9672, -1.7183) -> (-50.971, -1.7183)
  arc A14 (-40.6014, 30.8631) -> (-50.971, -1.7183) centre (0, 0) ccw
  line L3 (-40.6014, 30.8631) -> (-36.4403, 26.4027)
  arc A15 (-26.4027, -36.4403) -> (1.7183, -44.9672) centre (0, 0) ccw
  line L4 (1.7183, -44.9672) -> (1.7183, -50.971)
  arc A16 (-30.8631, -40.6014) -> (1.7183, -50.971) centre (0, 0) ccw
  line L5 (-30.8631, -40.6014) -> (-26.4027, -36.4403)
  arc A17 (36.4403, -26.4027) -> (44.9672, 1.7183) centre (0, 0) ccw
  line L6 (44.9672, 1.7183) -> (50.971, 1.7183)
  arc A18 (40.6014, -30.8631) -> (50.971, 1.7183) centre (0, 0) ccw
  line L7 (40.6014, -30.8631) -> (36.4403, -26.4027)
  spline S10 degree 3 poles (-5.3913, 45.3669) (-13.4446, 43.6223) (-19.3579, 41.2625) (-22.9312, 38.8101) (-25.0858, 37.3314) (-26.3571, 35.8297) (-26.8443, 34.5346) (-27.2279, 33.5151) (-27.1972, 32.632) (-26.744, 31.6708) (-26.7079, 31.5942) (-26.6688, 31.5172) (-26.6266, 31.4398) knots 0.061414 0.061414 0.061414 0.061414 0.474261 0.474261 0.474261 0.723202 0.723202 0.723202 0.919177 0.919177 0.919177 0.934786 0.934786 0.934786 0.934786
  arc A19 (-31.2084, 26.8976) -> (-31.4398, -26.6266) centre (0, 0) ccw
  spline S11 degree 3 poles (-31.2084, 26.8976) (-32.6199, 28.9795) (-33.0972, 31.2997) (-32.6861, 33.542) (-32.1693, 36.3616) (-30.3518, 39.0131) (-27.6472, 41.369) (-22.778, 45.6106) (-14.9399, 48.9827) (-5.4875, 50.4263) knots -0.97319 -0.97319 -0.97319 -0.97319 -0.77317 -0.77317 -0.77317 -0.521659 -0.521659 -0.521659 -0.068835 -0.068835 -0.068835 -0.068835
  spline S12 degree 3 poles (5.3913, -45.3669) (13.4446, -43.6223) (19.3579, -41.2625) (22.9312, -38.8101) (25.0858, -37.3314) (26.3571, -35.8297) (26.8443, -34.5346) (27.2279, -33.5151) (27.1972, -32.632) (26.744, -31.6708) (26.7079, -31.5942) (26.6688, -31.5172) (26.6266, -31.4398) knots 0.061414 0.061414 0.061414 0.061414 0.474261 0.474261 0.474261 0.723202 0.723202 0.723202 0.919177 0.919177 0.919177 0.934786 0.934786 0.934786 0.934786
  arc A20 (5.8105, -46.5038) -> (5.3913, -45.3669) centre (0, -48) ccw
  arc A21 (5.4875, -50.4263) -> (5.8891, -49.1482) centre (0, -48) ccw
  arc A22 (46.5038, 5.8105) -> (45.3669, 5.3913) centre (48, 0) ccw
  spline S13 degree 3 poles (45.3669, 5.3913) (43.6223, 13.4446) (41.2625, 19.3579) (38.8101, 22.9312) (37.3314, 25.0858) (35.8297, 26.3571) (34.5346, 26.8443) (33.5151, 27.2279) (32.632, 27.1972) (31.6708, 26.744) (31.5942, 26.7079) (31.5172, 26.6688) (31.4398, 26.6266) knots 0.061414 0.061414 0.061414 0.061414 0.474261 0.474261 0.474261 0.723202 0.723202 0.723202 0.919177 0.919177 0.919177 0.934786 0.934786 0.934786 0.934786
  arc A23 (31.2084, -26.8976) -> (31.4398, 26.6266) centre (0, 0) ccw
  spline S14 degree 3 poles (31.2084, -26.8976) (32.6199, -28.9795) (33.0972, -31.2997) (32.6861, -33.542) (32.1693, -36.3616) (30.3518, -39.0131) (27.6472, -41.369) (22.778, -45.6106) (14.9399, -48.9827) (5.4875, -50.4263) knots -0.97319 -0.97319 -0.97319 -0.97319 -0.77317 -0.77317 -0.77317 -0.521659 -0.521659 -0.521659 -0.068835 -0.068835 -0.068835 -0.068835
  arc A24 (50.4263, 5.4875) -> (49.1482, 5.8891) centre (48, 0) ccw
  arc A25 (26.8976, 31.2084) -> (-26.6266, 31.4398) centre (0, 0) ccw
  spline S15 degree 3 poles (26.8976, 31.2084) (28.9795, 32.6199) (31.2997, 33.0972) (33.542, 32.6861) (36.3616, 32.1693) (39.0131, 30.3518) (41.369, 27.6472) (45.6106, 22.778) (48.9827, 14.9399) (50.4263, 5.4875) knots -0.97319 -0.97319 -0.97319 -0.97319 -0.77317 -0.77317 -0.77317 -0.521659 -0.521659 -0.521659 -0.068835 -0.068835 -0.068835 -0.068835
  dimension "d201" = 60
  measures "d201" diameter of A10
extrude "Extrude29" cut sketch "Sketch21" against normal blind 1.2 contours A10 bodies 1
move_body "Move1" bodies 1 to x (-1, 0, 0) y (0, 1, 0) z (0, 0, -1) at (-121, 0, -4.8)
equation "hole_diameter = 109 mm"
equation "hole_wall_thinkness = 20 mm"
equation "button_thickness = 4 mm"
equation "button_diameter = 80 mm"
equation "d92 = button_diameter"
equation "d93 = button_thickness"
equation "d94 = button_thickness / 2"
equation "d95 = button_thickness * 2"
equation "d100 = button_thickness"
equation "d104 = button_thickness / 2"
equation "d105 = button_thickness * 1.5"
equation "d120 = button_thickness * 1.5"
equation "d124 = button_thickness * 1.5"
equation "d126 = button_diameter - button_thickness"
equation "d155 = hole_diameter"
equation "d156 = button_diameter + ( spacer * 2 )"
equation "spacer = 1.2 mm"
equation "d163 = -button_thickness * 1.5"
equation "d167 = spacer"
equation "d168 = spacer"
equation "d169 = spacer"
equation "d170 = spacer"
equation "d171 = spacer"
equation "d172 = spacer"
equation "d178 = spacer"
equation "d185 = button_thickness * 3"
equation "d186 = -button_thickness * 1.5"
equation "d190 = spacer * 5"
equation "d191 = -spacer"
equation "d195 = spacer * 2"
equation "d201 = button_diameter * 0.75"
equation "d202 = -spacer"
equation "d204 = spacer * 2.5"
equation "d205 = -d204"
equation "d206 = -spacer"
equation "d207 = spacer"
equation "d208 = spacer"
